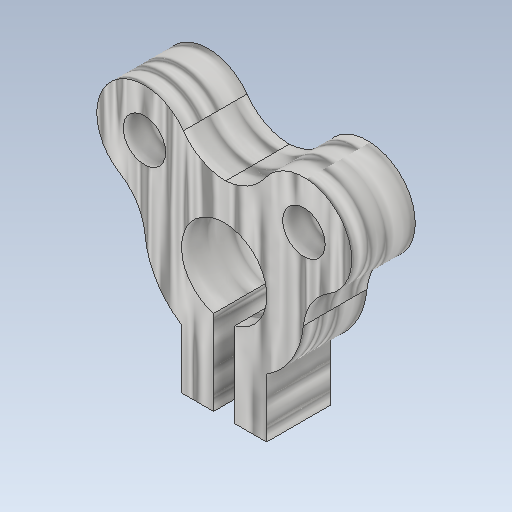
# Autodesk Inventor part: 横回転棒取り付けパーツ
Saved by Autodesk Inventor 2020 (Build 240168000, 168)
## iProperties
Created: 2019-09-03
Part Number: 横回転棒取り付けパーツ
Material: アルミニウム 7075
Document SubType Name: Modeling
Designer: tanjihayato
Density: 2.81 g/cm^3
Appearance: サテン - ブラシ仕上げ 重厚
Mass: 4.12874 g
Surface Area: 13.6392 cm^2
Volume: 1.4693 cm^3
Author: tanjihayato
Autodesk Inventor part; units mm, degrees
ref_plane "YZ Plane" through (0, 0, 0) normal (1, 0, 0) x (0, 1, 0)
ref_plane "XZ Plane" through (0, 0, 0) normal (0, 1, 0) x (-1, 0, 0)
ref_plane "XY Plane" through (0, 0, 0) normal (0, 0, 1) x (1, 0, 0)
sketch "スケッチ1" plane through (0, 0, 0) normal (0, 0, 1) x (1, 0, 0)
  circle A0 centre (0, 0) radius 4.025
  arc A1 (6.725498, 2.029361) -> (-6.725498, 2.029361) centre (0, 0) ccw
  line L0 (0, -11) -> (0, -19) construction
  line L1 (-3.025, -11) -> (-3.025, -19)
  line L2 (3.025, -19) -> (3.025, -11)
  arc A2 (3.025, -11) -> (-3.025, -11) centre (0, -11) ccw
  arc A3 (-3.025, -19) -> (3.025, -19) centre (0, -19) ccw
  arc A4 (-5.235739, -21.981218) -> (5.235739, -21.981218) centre (0, -19) ccw
  circle A5 centre (-7.525, -11) radius 1.25
  circle A6 centre (7.525, -11) radius 1.25
  line L3 (-7.525, -11) -> (7.525, -11) construction
  arc A7 (-11.411415, -8.73157) -> (-10.923603, -13.949491) centre (-7.525, -11) ccw
  arc A8 (-11.411415, -8.73157) -> (-6.725498, 2.029361) centre (-54.593809, 16.473208) ccw
  arc A9 (6.725498, 2.029361) -> (11.411415, -8.73157) centre (54.593809, 16.473208) ccw
  arc A10 (-5.235739, -21.981218) -> (-10.923603, -13.949491) centre (-48.685856, -46.721617) ccw
  arc A11 (10.923603, -13.949491) -> (5.235739, -21.981218) centre (48.685856, -46.721617) ccw
  arc A12 (10.923603, -13.949491) -> (11.411415, -8.73157) centre (7.525, -11) ccw
  point P0 (0, -15)
  dimension "d0" = 8.05
  dimension "d1" = 3
  dimension "d2" = 8
  dimension "d3" = 6.05
  dimension "d4" = 19
  dimension "d5" = 2.5
  dimension "d6" = 2.5
  dimension "d7" = 9
  dimension "d8" = 100
  dimension "d9" = 100
  dimension "d10" = 50
  dimension "d11" = 50
  dimension "d12" = 4.5
  dimension "d13" = 3
  constraints: 20 point on circle, 14 tangent, 13 centre point, 10 end point, 3 coincident, 3 point on line, 2 midpoint, 1 horizontal, 1 parallel, 1 vertical
  measures "d0" diameter of A0
  measures "d1" radial gap between concentric circles of A0 A1
  measures "d2" distance of L0.start L0.end
  measures "d3" diameter of A3
  measures "d4" distance of L0.end point (0, 0)
  measures "d5" diameter of A5
  measures "d6" diameter of A6
  measures "d7" diameter of A7
  measures "d8" diameter of A9
  measures "d9" diameter of A8
  measures "d10" radius of A11
  measures "d11" radius of A10
  measures "d12" radius of A12
  measures "d13" radial gap between concentric circles of A4 A3
sketch "スケッチ2" plane through (0, 0, 0) normal (0, 0, 1) x (1, 0, 0)
  circle A0 centre (-7.525, -11) radius 1.25 construction
  circle A1 centre (7.525, -11) radius 1.25 construction
  circle A2 centre (-7.525, -11) radius 2
  circle A3 centre (7.525, -11) radius 2
  arc A4 (-3.027118, -11.138035) -> (-7.062601, -15.47618) centre (-7.525, -11) ccw
  arc A5 (7.062601, -15.47618) -> (3.027118, -11.138035) centre (7.525, -11) ccw
  arc A6 (1, -21.898798) -> (-1, -21.898798) centre (0, -18) ccw
  line L0 (0, 0) -> (0, -18) construction
  line L1 (-1, -21.898798) -> (-1, -29.898798)
  line L2 (1, -21.898798) -> (1, -29.898798)
  line L3 (1, -29.898798) -> (4, -29.898798)
  line L4 (4, -29.898798) -> (4, -24.344289)
  line L5 (-1, -29.898798) -> (-4, -29.898798)
  line L6 (-4, -29.898798) -> (-4, -24.344289)
  arc A7 (-7.062601, -15.47618) -> (-4, -24.344289) centre (0, -18) ccw
  arc A8 (4, -24.344289) -> (7.062601, -15.47618) centre (0, -18) ccw
  arc A9 (3.027118, -11.138035) -> (-3.027118, -11.138035) centre (0, -18) ccw
  dimension "d14" = 4
  dimension "d15" = 4
  dimension "d16" = 9
  dimension "d17" = 9
  dimension "d18" = 8.05
  dimension "d19" = 18
  dimension "d20" = 8
  dimension "d21" = 8
  dimension "d22" = 2
  dimension "d23" = 1
  dimension "d24" = 3
  dimension "d25" = 3
  dimension "d27" = 7.5
  dimension "d28" = 7.5
  dimension "d29" = 7.5
  constraints: 14 end point, 12 point on circle, 8 centre point, 5 coincident, 3 vertical, 2 perpendicular, 1 horizontal, 1 point on line
  measures "d14" diameter of A2
  measures "d15" diameter of A3
  measures "d16" diameter of A4
  measures "d17" diameter of A5
  measures "d18" diameter of A6
  measures "d19" distance of L0.start L0.end
  measures "d20" distance of L1.start L1.end
  measures "d21" distance of L2.start L2.end
  measures "d22" distance between parallel lines of L1 L2
  measures "d23" distance between parallel lines of L2 L0
  measures "d24" distance of L2.end L3.end
  measures "d25" distance of L1.end L5.end
  measures "d27" radius of A9
  measures "d28" radius of A7
  measures "d29" radius of A8
sketch "スケッチ2 outline for 押し出し1" plane through (0, 0, 0) normal (0, 0, 1) x (1, 0, 0)
  line L0 (-1, -29.898798) -> (-1, -21.898798)
  line L1 (-4, -29.898798) -> (-1, -29.898798)
  arc A0 (-1, -21.898798) -> (1, -21.898798) centre (0, -18) cw
  line L2 (-4, -24.344289) -> (-4, -29.898798)
  line L3 (1, -21.898798) -> (1, -29.898798)
  arc A1 (-7.062601, -15.47618) -> (-4, -24.344289) centre (0, -18) ccw
  line L4 (1, -29.898798) -> (4, -29.898798)
  arc A2 (-3.027118, -11.138035) -> (-7.062601, -15.47618) centre (-7.525, -11) ccw
  line L5 (4, -29.898798) -> (4, -24.344289)
  arc A3 (3.027118, -11.138035) -> (-3.027118, -11.138035) centre (0, -18) ccw
  arc A4 (4, -24.344289) -> (7.062601, -15.47618) centre (0, -18) ccw
  arc A5 (7.062601, -15.47618) -> (3.027118, -11.138035) centre (7.525, -11) ccw
  circle A6 centre (-7.525, -11) radius 2
  circle A7 centre (7.525, -11) radius 2
extrude "押し出し1" add sketch "スケッチ2 outline for 押し出し1" along normal blind 6
fillet "フィレット1" radius 5 4 edges at (-3.0271, -11.138, 3) (3.0271, -11.138, 3) (7.0626, -15.4762, 3) (-7.0626, -15.4762, 3)
equation "\"d21\" = d20"
